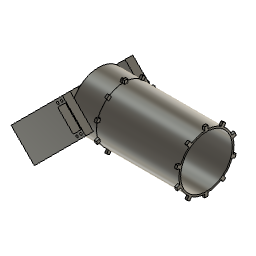
Cannon (Autodesk Fusion 360 archive; units mm, degrees)
design "Cannon" references "FeeTech FS5109M Metal Gear Servo Outer volume", "mg995"
Autodesk Fusion 360 part; units mm, degrees
sketch "Sketch1" plane through (0, 0, 0) normal (1, 0, 0) x (0, 1, 0)
  circle A0 centre (0, 0) radius 50
  circle A1 centre (0, 0) radius 47
  dimension "d1" = 94
  constraint coincident A0.centre A1.centre
  measures "d1" diameter of A1
extrude "Extrude1" add sketch "Sketch1" along normal blind 150 makes body 1
sketch "Sketch2" plane through (150, 0, 0) normal (1, 0, 0) x (0, 1, 0)
  circle A0 centre (0, 0) radius 47
  circle A1 centre (0, 0) radius 50
  line L0 (3, 49.9099) -> (-3, 49.9099)
  line L1 (-3, 49.9099) -> (-3, 55.9099)
  line L2 (-3, 55.9099) -> (3, 55.9099)
  line L3 (3, 55.9099) -> (3, 49.9099)
  line L4 (-35.2901, 43.4687) -> (-30.436, 46.9954)
  line L5 (-31.7634, 38.6146) -> (-35.2901, 43.4687)
  line L6 (-26.9093, 42.1413) -> (-31.7634, 38.6146)
  line L7 (-30.436, 46.9954) -> (-26.9093, 42.1413)
  line L8 (-54.1005, 14.4239) -> (-52.2464, 20.1303)
  line L9 (-48.3942, 12.5698) -> (-54.1005, 14.4239)
  line L10 (-46.5401, 18.2762) -> (-48.3942, 12.5698)
  line L11 (-52.2464, 20.1303) -> (-46.5401, 18.2762)
  line L12 (-52.2464, -20.1303) -> (-54.1005, -14.4239)
  line L13 (-46.5401, -18.2762) -> (-52.2464, -20.1303)
  line L14 (-48.3942, -12.5698) -> (-46.5401, -18.2762)
  line L15 (-54.1005, -14.4239) -> (-48.3942, -12.5698)
  line L16 (-30.436, -46.9954) -> (-35.2901, -43.4687)
  line L17 (-26.9093, -42.1413) -> (-30.436, -46.9954)
  line L18 (-31.7634, -38.6146) -> (-26.9093, -42.1413)
  line L19 (-35.2901, -43.4687) -> (-31.7634, -38.6146)
  line L20 (3, -55.9099) -> (-3, -55.9099)
  line L21 (3, -49.9099) -> (3, -55.9099)
  line L22 (-3, -49.9099) -> (3, -49.9099)
  line L23 (-3, -55.9099) -> (-3, -49.9099)
  line L24 (35.2901, -43.4687) -> (30.436, -46.9954)
  line L25 (31.7634, -38.6146) -> (35.2901, -43.4687)
  line L26 (26.9093, -42.1413) -> (31.7634, -38.6146)
  line L27 (30.436, -46.9954) -> (26.9093, -42.1413)
  line L28 (54.1005, -14.4239) -> (52.2464, -20.1303)
  line L29 (48.3942, -12.5698) -> (54.1005, -14.4239)
  line L30 (46.5401, -18.2762) -> (48.3942, -12.5698)
  line L31 (52.2464, -20.1303) -> (46.5401, -18.2762)
  line L32 (52.2464, 20.1303) -> (54.1005, 14.4239)
  line L33 (46.5401, 18.2762) -> (52.2464, 20.1303)
  line L34 (48.3942, 12.5698) -> (46.5401, 18.2762)
  line L35 (54.1005, 14.4239) -> (48.3942, 12.5698)
  line L36 (30.436, 46.9954) -> (35.2901, 43.4687)
  line L37 (26.9093, 42.1413) -> (30.436, 46.9954)
  line L38 (31.7634, 38.6146) -> (26.9093, 42.1413)
  line L39 (35.2901, 43.4687) -> (31.7634, 38.6146)
  dimension "d4" = 6
  dimension "d5" = 6
  dimension "d7" = 360
  constraint horizontal L0
  constraint vertical L1
  constraint horizontal L2
  constraint vertical L3
  constraint coincident A1 L0.start
  measures "d4" distance of L0.start L0.end
  measures "d5" distance of L0.start L2.end
extrude "Extrude2" add sketch "Sketch2" against normal blind 4 contours A1 L32 L33 L35 | A1 L28 L29 L31 | A1 L36 L37 L39 | A1 L24 L25 L27 | A1 L1 L2 L3 | A1 L20 L21 L23 | A1 L4 L5 L7 | A1 L16 L17 L19 | A1 L8 L9 L11 | A1 L12 L13 L15 bodies 1
sketch "Sketch3" plane through (0, 0, 0) normal (-1, 0, 0) x (0, -1, 0)
  circle A0 centre (0, 0) radius 47
  circle A1 centre (0, 0) radius 50
  line L0 (3, 49.9099) -> (-3, 49.9099)
  line L1 (-3, 49.9099) -> (-3, 55.9099)
  line L2 (-3, 55.9099) -> (3, 55.9099)
  line L3 (3, 55.9099) -> (3, 49.9099)
  line L4 (-35.2901, 43.4687) -> (-30.436, 46.9954)
  line L5 (-31.7634, 38.6146) -> (-35.2901, 43.4687)
  line L6 (-26.9093, 42.1413) -> (-31.7634, 38.6146)
  line L7 (-30.436, 46.9954) -> (-26.9093, 42.1413)
  line L8 (-54.1005, 14.4239) -> (-52.2464, 20.1303)
  line L9 (-48.3942, 12.5698) -> (-54.1005, 14.4239)
  line L10 (-46.5401, 18.2762) -> (-48.3942, 12.5698)
  line L11 (-52.2464, 20.1303) -> (-46.5401, 18.2762)
  line L12 (-52.2464, -20.1303) -> (-54.1005, -14.4239)
  line L13 (-46.5401, -18.2762) -> (-52.2464, -20.1303)
  line L14 (-48.3942, -12.5698) -> (-46.5401, -18.2762)
  line L15 (-54.1005, -14.4239) -> (-48.3942, -12.5698)
  line L16 (-30.436, -46.9954) -> (-35.2901, -43.4687)
  line L17 (-26.9093, -42.1413) -> (-30.436, -46.9954)
  line L18 (-31.7634, -38.6146) -> (-26.9093, -42.1413)
  line L19 (-35.2901, -43.4687) -> (-31.7634, -38.6146)
  line L20 (3, -55.9099) -> (-3, -55.9099)
  line L21 (3, -49.9099) -> (3, -55.9099)
  line L22 (-3, -49.9099) -> (3, -49.9099)
  line L23 (-3, -55.9099) -> (-3, -49.9099)
  line L24 (35.2901, -43.4687) -> (30.436, -46.9954)
  line L25 (31.7634, -38.6146) -> (35.2901, -43.4687)
  line L26 (26.9093, -42.1413) -> (31.7634, -38.6146)
  line L27 (30.436, -46.9954) -> (26.9093, -42.1413)
  line L28 (54.1005, -14.4239) -> (52.2464, -20.1303)
  line L29 (48.3942, -12.5698) -> (54.1005, -14.4239)
  line L30 (46.5401, -18.2762) -> (48.3942, -12.5698)
  line L31 (52.2464, -20.1303) -> (46.5401, -18.2762)
  line L32 (52.2464, 20.1303) -> (54.1005, 14.4239)
  line L33 (46.5401, 18.2762) -> (52.2464, 20.1303)
  line L34 (48.3942, 12.5698) -> (46.5401, 18.2762)
  line L35 (54.1005, 14.4239) -> (48.3942, 12.5698)
  line L36 (30.436, 46.9954) -> (35.2901, 43.4687)
  line L37 (26.9093, 42.1413) -> (30.436, 46.9954)
  line L38 (31.7634, 38.6146) -> (26.9093, 42.1413)
  line L39 (35.2901, 43.4687) -> (31.7634, 38.6146)
  dimension "d10" = 6
  dimension "d12" = 360
  constraint horizontal L0
  constraint vertical L1
  constraint horizontal L2
  constraint vertical L3
  constraint coincident A1 L0.start
  measures "d10" distance of L0.start L2.end
extrude "Extrude3" add sketch "Sketch3" against normal blind 4 contours A1 L32 L33 L35 | A1 L28 L29 L31 | A1 L36 L37 L39 | A1 L24 L25 L27 | A1 L1 L2 L3 | A1 L20 L21 L23 | A1 L4 L5 L7 | A1 L16 L17 L19 | A1 L8 L9 L11 | A1 L12 L13 L15 bodies 1
extrude "Extrude4" add sketch "Sketch1" along normal blind 3 contours A1 bodies 1
extrude "Extrude5" add sketch "Sketch1" against normal blind 60 separate body makes body 2
sketch "Sketch4" plane through (0, 0, 0) normal (-1, 0, 0) x (0, -1, 0)
  arc A0 (-46.5401, -18.2762) -> (-31.7634, -38.6146) centre (0, 0) ccw
  line L0 (-31.7634, -38.6146) -> (-35.2901, -43.4687)
  line L1 (-35.2901, -43.4687) -> (-30.436, -46.9954)
  line L2 (-30.436, -46.9954) -> (-26.9093, -42.1413)
  arc A1 (-26.9093, -42.1413) -> (-3, -49.9099) centre (0, 0) ccw
  line L3 (-3, -49.9099) -> (-3, -55.9099)
  line L4 (-3, -55.9099) -> (3, -55.9099)
  line L5 (3, -55.9099) -> (3, -49.9099)
  arc A2 (3, -49.9099) -> (26.9093, -42.1413) centre (0, 0) ccw
  line L6 (26.9093, -42.1413) -> (30.436, -46.9954)
  line L7 (30.436, -46.9954) -> (35.2901, -43.4687)
  line L8 (35.2901, -43.4687) -> (31.7634, -38.6146)
  arc A3 (31.7634, -38.6146) -> (46.5401, -18.2762) centre (0, 0) ccw
  line L9 (46.5401, -18.2762) -> (52.2464, -20.1303)
  line L10 (52.2464, -20.1303) -> (54.1005, -14.4239)
  line L11 (54.1005, -14.4239) -> (48.3942, -12.5698)
  arc A4 (48.3942, -12.5698) -> (48.3942, 12.5698) centre (0, 0) ccw
  line L12 (48.3942, 12.5698) -> (54.1005, 14.4239)
  line L13 (54.1005, 14.4239) -> (52.2464, 20.1303)
  line L14 (52.2464, 20.1303) -> (46.5401, 18.2762)
  arc A5 (46.5401, 18.2762) -> (31.7634, 38.6146) centre (0, 0) ccw
  line L15 (31.7634, 38.6146) -> (35.2901, 43.4687)
  line L16 (35.2901, 43.4687) -> (30.436, 46.9954)
  line L17 (30.436, 46.9954) -> (26.9093, 42.1413)
  arc A6 (26.9093, 42.1413) -> (3, 49.9099) centre (0, 0) ccw
  line L18 (3, 49.9099) -> (3, 55.9099)
  line L19 (3, 55.9099) -> (-3, 55.9099)
  line L20 (-3, 55.9099) -> (-3, 49.9099)
  arc A7 (-3, 49.9099) -> (-26.9093, 42.1413) centre (0, 0) ccw
  line L21 (-26.9093, 42.1413) -> (-30.436, 46.9954)
  line L22 (-30.436, 46.9954) -> (-35.2901, 43.4687)
  line L23 (-35.2901, 43.4687) -> (-31.7634, 38.6146)
  arc A8 (-31.7634, 38.6146) -> (-46.5401, 18.2762) centre (0, 0) ccw
  line L24 (-46.5401, 18.2762) -> (-52.2464, 20.1303)
  line L25 (-52.2464, 20.1303) -> (-54.1005, 14.4239)
  line L26 (-54.1005, 14.4239) -> (-48.3942, 12.5698)
  arc A9 (-48.3942, 12.5698) -> (-48.3942, -12.5698) centre (0, 0) ccw
  line L27 (-48.3942, -12.5698) -> (-54.1005, -14.4239)
  line L28 (-54.1005, -14.4239) -> (-52.2464, -20.1303)
  line L29 (-52.2464, -20.1303) -> (-46.5401, -18.2762)
  line L30 (-3, 49.9099) -> (0, 55.9099)
  line L31 (0, 55.9099) -> (3, 49.9099)
  line L32 (3, 49.9099) -> (-3, 49.9099)
  constraint coincident L20.end A7.start
  constraint midpoint L19 L30.end
  constraint coincident A6.end L18.start
move_body "Move1" bodies 1 to x (1, 0, 0) y (0, 1, 0) z (0, 0, 1) at (0, 0, -90)
extrude "Extrude6" add sketch "Sketch4" along normal blind 4 contours L30 L31 L32 bodies 2
move_body "Move2" bodies 1 to x (1, 0, 0) y (0, 1, 0) z (0, 0, 1) at (0, 0, 90)
sketch "Sketch5" plane through (0, 0, 0) normal (-1, 0, 0) x (0, -1, 0)
  arc A0 (-46.5401, -18.2762) -> (-31.7634, -38.6146) centre (0, 0) ccw
  line L0 (-31.7634, -38.6146) -> (-35.2901, -43.4687)
  line L1 (-35.2901, -43.4687) -> (-30.436, -46.9954)
  line L2 (-30.436, -46.9954) -> (-26.9093, -42.1413)
  arc A1 (-26.9093, -42.1413) -> (-3, -49.9099) centre (0, 0) ccw
  line L3 (-3, -49.9099) -> (-3, -55.9099)
  line L4 (-3, -55.9099) -> (3, -55.9099)
  line L5 (3, -55.9099) -> (3, -49.9099)
  arc A2 (3, -49.9099) -> (26.9093, -42.1413) centre (0, 0) ccw
  line L6 (26.9093, -42.1413) -> (30.436, -46.9954)
  line L7 (30.436, -46.9954) -> (35.2901, -43.4687)
  line L8 (35.2901, -43.4687) -> (31.7634, -38.6146)
  arc A3 (31.7634, -38.6146) -> (46.5401, -18.2762) centre (0, 0) ccw
  line L9 (46.5401, -18.2762) -> (52.2464, -20.1303)
  line L10 (52.2464, -20.1303) -> (54.1005, -14.4239)
  line L11 (54.1005, -14.4239) -> (48.3942, -12.5698)
  arc A4 (48.3942, -12.5698) -> (48.3942, 12.5698) centre (0, 0) ccw
  line L12 (48.3942, 12.5698) -> (54.1005, 14.4239)
  line L13 (54.1005, 14.4239) -> (52.2464, 20.1303)
  line L14 (52.2464, 20.1303) -> (46.5401, 18.2762)
  arc A5 (46.5401, 18.2762) -> (31.7634, 38.6146) centre (0, 0) ccw
  line L15 (31.7634, 38.6146) -> (35.2901, 43.4687)
  line L16 (35.2901, 43.4687) -> (30.436, 46.9954)
  line L17 (30.436, 46.9954) -> (26.9093, 42.1413)
  arc A6 (26.9093, 42.1413) -> (3, 49.9099) centre (0, 0) ccw
  line L18 (3, 49.9099) -> (3, 55.9099)
  line L19 (3, 55.9099) -> (-3, 55.9099)
  line L20 (-3, 55.9099) -> (-3, 49.9099)
  arc A7 (-3, 49.9099) -> (-26.9093, 42.1413) centre (0, 0) ccw
  line L21 (-26.9093, 42.1413) -> (-30.436, 46.9954)
  line L22 (-30.436, 46.9954) -> (-35.2901, 43.4687)
  line L23 (-35.2901, 43.4687) -> (-31.7634, 38.6146)
  arc A8 (-31.7634, 38.6146) -> (-46.5401, 18.2762) centre (0, 0) ccw
  line L24 (-46.5401, 18.2762) -> (-52.2464, 20.1303)
  line L25 (-52.2464, 20.1303) -> (-54.1005, 14.4239)
  line L26 (-54.1005, 14.4239) -> (-48.3942, 12.5698)
  arc A9 (-48.3942, 12.5698) -> (-48.3942, -12.5698) centre (0, 0) ccw
  line L27 (-48.3942, -12.5698) -> (-54.1005, -14.4239)
  line L28 (-54.1005, -14.4239) -> (-52.2464, -20.1303)
  line L29 (-52.2464, -20.1303) -> (-46.5401, -18.2762)
  circle A10 centre (0, 0) radius 1.5
  dimension "d27" = 3
  constraint coincident A0.centre A1.centre
  measures "d27" diameter of A10
extrude "Extrude7" cut sketch "Sketch5" against normal blind 1 contours A10 bodies 1
sketch "Sketch6" plane through (-41.4, 0, 0) normal (-1, 0, 0) x (0, -1, 0)
  line L0 (-6.05, 9.55) -> (-6.05, 7.55)
  arc A0 (-7.55, 6.05) -> (-6.05, 7.55) centre (-7.55, 7.55) ccw
  line L1 (-7.55, 6.05) -> (-9.55, 6.05)
  line L2 (-9.55, 6.05) -> (-9.55, -26.75)
  line L3 (-9.55, -26.75) -> (-7.55, -26.75)
  arc A1 (-6.05, -28.25) -> (-7.55, -26.75) centre (-7.55, -28.25) ccw
  line L4 (-6.05, -28.25) -> (-6.05, -30.25)
  line L5 (-6.05, -30.25) -> (6.05, -30.25)
  line L6 (6.05, -30.25) -> (6.05, -28.25)
  arc A2 (7.55, -26.75) -> (6.05, -28.25) centre (7.55, -28.25) ccw
  line L7 (7.55, -26.75) -> (9.55, -26.75)
  line L8 (9.55, -26.75) -> (9.55, 6.05)
  line L9 (9.55, 6.05) -> (7.55, 6.05)
  arc A3 (6.05, 7.55) -> (7.55, 6.05) centre (7.55, 7.55) ccw
  line L10 (6.05, 7.55) -> (6.05, 9.55)
  line L11 (6.05, 9.55) -> (-6.05, 9.55)
  line L12 (-90, 80) -> (102.9005, 80)
  line L13 (102.9005, 80) -> (102.9005, -93.0989)
  line L14 (102.9005, -93.0989) -> (-90, -93.0989)
  line L15 (-90, -93.0989) -> (-90, 80)
  constraint horizontal L12
  constraint vertical L13
  constraint horizontal L14
  constraint vertical L15
extrude "Extrude8" cut sketch "Sketch6" against normal blind 280 keep common part bodies 1 2
move_body "Move3" bodies 1 to x (1, 0, 0) y (0, 1, 0) z (0, 0, 1) at (0, 0, 115)
move_body "Move4" bodies 1 to x (1, 0, 0) y (0, 1, 0) z (0, 0, 1) at (0, 0, -115)
extrude "Extrude9" add sketch "Sketch1" along normal blind 3 contours A1 bodies 1
extrude "Extrude10" cut sketch "Sketch5" against normal blind 1 contours A10 bodies 1
extrude "Extrude11" add 1 faces at (-41.4, 48.8138, -2.484) along direction (-1, 0, 0) blind 5 on bodies 2 bodies 2
sketch "Sketch7" plane through (-46.4, 0, 0) normal (-1, 0, 0) x (0, -1, 0)
  circle A0 centre (0, 0) radius 47
  circle A1 centre (0, 0) radius 50
  circle A2 centre (0, 0) radius 47
  constraint coincident A0.centre A1.centre
extrude "Extrude12" add sketch "Sketch7" against normal blind 4 contours A0 A2 bodies 2
sketch "Sketch8" plane through (-46.4, 0, 0) normal (-1, 0, 0) x (0, -1, 0)
  circle A0 centre (0, 0) radius 50
  line L0 (-40, 20) -> (-25, 20)
  line L1 (-25, 20) -> (-25, -20)
  line L2 (-25, -20) -> (-40, -20)
  line L3 (-40, -20) -> (-40, 20)
  dimension "d50" = 15
  dimension "d51" = 40
  constraint horizontal L0
  constraint vertical L1
  constraint horizontal L2
  constraint vertical L3
  measures "d50" distance of L0.start L0.end
  measures "d51" distance of L0.start L2.end
extrude "Extrude13" cut sketch "Sketch8" against normal blind 10 contours L0 L1 L2 L3 bodies 2
sketch "Sketch9" plane through (-14.6, 0, 0) normal (-1, 0, 0) x (0, -1, 0)
  arc A0 (9.35, 9.8189) -> (8.55, 10.05) centre (8.55, 8.55) ccw
  line L0 (9.35, 9.8189) -> (9.35, 15.45)
  arc A1 (9.35, 15.45) -> (7.85, 16.95) centre (7.85, 15.45) ccw
  line L1 (7.85, 16.95) -> (6.25, 16.95)
  line L2 (6.25, 16.95) -> (6.25, 16.2708)
  arc A2 (3.75, 16.2708) -> (6.25, 16.2708) centre (5, 14.4) ccw
  line L3 (3.75, 16.2708) -> (3.75, 16.95)
  line L4 (3.75, 16.95) -> (-3.75, 16.95)
  line L5 (-3.75, 16.95) -> (-3.75, 16.2708)
  arc A3 (-6.25, 16.2708) -> (-3.75, 16.2708) centre (-5, 14.4) ccw
  line L6 (-6.25, 16.2708) -> (-6.25, 16.95)
  line L7 (-6.25, 16.95) -> (-7.85, 16.95)
  arc A4 (-7.85, 16.95) -> (-9.35, 15.45) centre (-7.85, 15.45) ccw
  line L8 (-9.35, 15.45) -> (-9.35, 9.8189)
  arc A5 (-8.55, 10.05) -> (-9.35, 9.8189) centre (-8.55, 8.55) ccw
  line L9 (-8.55, 10.05) -> (8.55, 10.05)
  line L10 (-9.35, 10.9766) -> (9.35, 10.9766)
  line L11 (9.35, 10.9766) -> (9.35, 69.9703)
  line L12 (9.35, 69.9703) -> (-9.35, 69.9703)
  line L13 (-9.35, 69.9703) -> (-9.35, 10.9766)
  line L14 (-9.35, -31.9165) -> (9.35, -31.9165)
  line L15 (9.35, -31.9165) -> (9.35, -86.2684)
  line L16 (9.35, -86.2684) -> (-9.35, -86.2684)
  line L17 (-9.35, -86.2684) -> (-9.35, -31.9165)
  circle A6 centre (-5, 14.4) radius 2.25
  circle A7 centre (5, 14.4) radius 2.25
  circle A8 centre (5, -35) radius 2.2361
  circle A9 centre (-5, -35) radius 2.2361
  constraint horizontal L10
  constraint vertical L11
  constraint horizontal L12
  constraint vertical L13
  constraint coincident L8 L10.start
  constraint horizontal L14
  constraint vertical L15
  constraint horizontal L16
  constraint vertical L17
  constraint concentric A3 A6
  constraint concentric A2 A7
extrude "Extrude14" add sketch "Sketch9" along normal blind 5 contours L0 A1 L1 L2 A2 L3 L4 L5 A3 L6 L7 A4 L8 L10 L11 L13 A6 A7 | A1 L1 L2 L3 L4 L5 L6 L7 A4 L11 L12 L13 A6 A7 | L14 L15 L16 L17 bodies 2
extrude "Extrude15" cut 2 faces at (-14.6, 1.0444, 63.2808) (-14.6, 1.0444, -74.1462) along direction (-1, 0, 0) blind 10 on bodies 2 bodies 2
ref_plane "WorkPlane1" through (0, -50, 0) normal (0, 1, 0) x (0, 0, 1)
sketch "Sketch10" plane through (0, -50, 0) normal (0, 1, 0) x (1, 0, 0)
  line L0 (0, 0) -> (-42.4264, -42.4264)
  line L1 (0, 0) -> (60, 0) construction
  line L2 (-42.4264, -42.4264) -> (-148.4924, 63.6396)
  line L3 (-148.4924, 63.6396) -> (-106.066, 106.066)
  line L4 (-106.066, 106.066) -> (0, 0)
  circle A0 centre (-28.2843, 0) radius 1
  point P0 (-28.2843, 0)
  dimension "d59" = 135
  dimension "d60" = 60
  dimension "d61" = 150
  dimension "d62" = 60
  dimension "d81" = 2
  constraint horizontal L1
  constraint coincident L0.start L1.start
  constraint perpendicular L0 L2
  constraint perpendicular L2 L3
  constraint coincident P0 A0.centre
  measures "d59" angle of L0 L1
  measures "d60" distance of L0.start L0.end
  measures "d61" distance of L0.end L2.end
  measures "d62" distance of L2.end L3.end
  measures "d81" diameter of A0
extrude "Extrude16" add sketch "Sketch10" against normal blind 14 separate body contours L0 L2 L3 L4 | A0 makes body 3
sketch "Sketch11" plane through (0, -58, 0) normal (0, 1, 0) x (-1, 0, 0)
  arc A0 (25.0025, 9.4462) -> (21.2132, 7.0711) centre (28.2843, 0) ccw
  line L0 (25.0025, 9.4462) -> (39.2444, 23.6881)
  line L1 (39.2444, 23.6881) -> (51.9723, 10.9602)
  line L2 (51.9723, 10.9602) -> (37.7304, -3.2818)
  arc A1 (35.3553, -7.0711) -> (37.7304, -3.2818) centre (28.2843, 0) ccw
  line L3 (35.3553, -7.0711) -> (56.5685, 14.1421)
  line L4 (56.5685, 14.1421) -> (42.4264, 28.2843)
  line L5 (42.4264, 28.2843) -> (21.2132, 7.0711)
sketch "Sketch12" plane through (0, -58, 0) normal (0, 1, 0) x (-1, 0, 0)
  line L0 (42.4264, 28.2841) -> (14.1421, -0.0002)
  line L1 (42.4264, 28.2841) -> (82.4264, 28.2841) construction
  line L2 (14.1421, -0.0002) -> (28.2842, -14.1423)
  line L3 (28.2842, -14.1423) -> (56.5685, 14.142)
  line L4 (56.5685, 14.142) -> (42.4264, 28.2841)
  dimension "d70" = 135
  dimension "d71" = 40
  constraint horizontal L1
  constraint perpendicular L0 L2
  constraint perpendicular L2 L3
  constraint perpendicular L0 L4
  measures "d70" angle of L0 L1
  measures "d71" distance of L0.start L0.end
extrude "Extrude17" cut sketch "Sketch12" along normal blind 10 and the other way blind 9 bodies 3
sketch "Sketch13" plane through (0, -66.5, 0) normal (0, -1, 0) x (1, 0, 0)
  arc A0 (-51.4134, 28.786) -> (-49.9992, 30.2002) centre (-49.3207, 28.1075) ccw
  line L0 (-51.4134, 28.786) -> (-51.6188, 28.9914)
  line L1 (-51.6188, 28.9914) -> (-57.2756, 23.3345)
  line L2 (-57.2756, 23.3345) -> (-57.0703, 23.1292)
  arc A1 (-58.4845, 21.715) -> (-57.0703, 23.1292) centre (-56.3918, 21.0364) ccw
  line L3 (-58.4845, 21.715) -> (-58.6899, 21.9203)
  line L4 (-58.6899, 21.9203) -> (-61.5183, 19.0919)
  line L5 (-61.5183, 19.0919) -> (-56.5685, 14.1421)
  line L6 (-56.5685, 14.1421) -> (-42.4264, 28.2843)
  line L7 (-42.4264, 28.2843) -> (-47.3762, 33.234)
  line L8 (-47.3762, 33.234) -> (-50.2046, 30.4056)
  line L9 (-50.2046, 30.4056) -> (-49.9992, 30.2002)
  circle A2 centre (-49.3207, 28.1075) radius 2.2
  circle A3 centre (-56.3918, 21.0364) radius 2.2
  line L10 (-17.6815, -3.5317) -> (-14.3227, -6.8905)
  circle A4 centre (-14.3227, -6.8905) radius 2.2
  circle A5 centre (-21.3938, -13.9615) radius 2.2
  dimension "d76" = 4.75
  dimension "d77" = 4.4
  dimension "d78" = 4.4
  constraint concentric A0 A2
  constraint concentric A1 A3
  constraint coincident L10.end A4.centre
  measures "d76" distance of L10.start L10.end
  measures "d77" diameter of A4
  measures "d78" diameter of A5
extrude "Extrude18" cut sketch "Sketch13" against normal blind 30 contours A0 A2 | A1 A3 | A4 | A5 bodies 3
extrude "Extrude19" cut sketch "Sketch10" along normal blind 1 contours A0 bodies 2
sketch "Sketch14" plane through (0, -50, 0) normal (0, 1, 0) x (-1, 0, 0)
  circle A0 centre (56.3918, 21.0364) radius 2.2
  circle A1 centre (14.3227, -6.8905) radius 2.2
  circle A2 centre (49.3207, 28.1075) radius 2.2
  circle A3 centre (21.3938, -13.9615) radius 2.2
  line L0 (106.066, -106.066) -> (148.4924, -63.6396)
  line L1 (148.4924, -63.6396) -> (42.4264, 42.4264)
  line L2 (42.4264, 42.4264) -> (0, 0)
  line L3 (0, 0) -> (106.066, -106.066)
  line L4 (134.3503, -49.4975) -> (91.9239, -91.9239)
  line L5 (56.5685, 14.142) -> (28.2842, -14.1423)
  line L6 (28.2842, -14.1423) -> (14.1421, -0.0002)
  line L7 (14.1421, -0.0002) -> (42.4264, 28.2841)
  line L8 (42.4264, 28.2841) -> (56.5685, 14.142)
  dimension "d84" = 20
  constraint coincident L3 L4.end
  constraint perpendicular L3 L4
  measures "d84" distance of L0.end L4.start
extrude "Extrude20" add sketch "Sketch14" along normal blind 114 contours L0 L1 L3 L4 bodies 3
sketch "Sketch15" plane through (-91.9239, 0, -91.9239) normal (0.707107, 0, 0.707107) x (0, 1, 0)
  line L0 (-50, 60) -> (-50, 0)
  line L1 (-50, 0) -> (64, 0)
  line L2 (64, 0) -> (64, 60)
  line L3 (64, 60) -> (-50, 60)
  line L4 (50, 0) -> (50, 60)
  dimension "d87" = 14
  constraint coincident L3 L4.end
  constraint perpendicular L3 L4
  measures "d87" distance of L1.end L4.start
extrude "Extrude21" add sketch "Sketch15" along normal blind 122 contours L1 L2 L3 L4 bodies 3
move_face "OffsetFaces1" offset -8 1 faces at (-14.1421, -54.6667, 14.1421) on bodies 3
ref_plane "WorkPlane2" through (0, 50, 0) normal (0, 1, 0) x (0, 0, 1)
sketch "Sketch16" plane through (0, 50, 0) normal (0, 1, 0) x (1, 0, 0)
  circle A0 centre (-28.2, 0) radius 5
  dimension "d92" = 28.2
  dimension "d93" = 10
  measures "d92" distance of origin A0.centre
  measures "d93" diameter of A0
extrude "Extrude22" cut sketch "Sketch16" along normal blind 20 and the other way blind 10 bodies 2 3
sketch "Sketch17" plane through (-91.9239, 0, -91.9239) normal (0.707107, 0, 0.707107) x (0, 1, 0)
  line L0 (50, 0) -> (50, 60)
  line L1 (50, 60) -> (-50, 60)
  line L2 (-50, 60) -> (-50, 0)
  line L3 (-50, 0) -> (50, 0)
move_face "OffsetFaces2" offset -10 1 faces at (-120.2082, -21.3333, -91.9239) on bodies 3
sketch "Sketch18" plane through (-91.9239, 0, -91.9239) normal (0.707107, 0, 0.707107) x (0, 1, 0)
  circle A0 centre (-30, 50) radius 1.9
  circle A1 centre (0, 50) radius 1.9
  circle A2 centre (30, 50) radius 1.9
  circle A3 centre (-30, 10) radius 1.9
  circle A4 centre (0, 10) radius 1.9
  circle A5 centre (30, 10) radius 1.9
  dimension "d99" = 3.8
  dimension "d100" = 3.8
  dimension "d101" = 3.8
  dimension "d102" = 3.8
  dimension "d103" = 3.8
  dimension "d104" = 3.8
  measures "d99" diameter of A0
  measures "d100" diameter of A1
  measures "d101" diameter of A2
  measures "d102" diameter of A3
  measures "d103" diameter of A4
  measures "d104" diameter of A5
extrude "Extrude23" cut sketch "Sketch18" against normal blind 40 bodies 3
copy_body "Body->Comp1" bodies 1 removing the originals makes body 4 in component "Barrel"
copy_body "Body->Comp2" bodies 2 removing the originals makes body 5 in component "Base"
copy_body "Body->Comp3" bodies 3 removing the originals makes body 6 in component "Support"
move_face "OffsetFaces1'" offset -2 2 faces at (-14.6, -1.0317, 26.6651) (-14.6, 1.0451, -40.1306) on bodies 5 in component "Base"
sketch "Sketch19" plane through (0, 0, 0) normal (-1, 0, 0) x (0, -1, 0)
  circle A0 centre (0, 0) radius 1.5
  arc A1 (-46.5401, -18.2762) -> (-31.7634, -38.6146) centre (0, 0) ccw
  line L0 (-31.7634, -38.6146) -> (-35.2901, -43.4687)
  line L1 (-35.2901, -43.4687) -> (-30.436, -46.9954)
  line L2 (-30.436, -46.9954) -> (-26.9093, -42.1413)
  arc A2 (-26.9093, -42.1413) -> (-3, -49.9099) centre (0, 0) ccw
  line L3 (-3, -49.9099) -> (-3, -55.9099)
  line L4 (-3, -55.9099) -> (3, -55.9099)
  line L5 (3, -55.9099) -> (3, -49.9099)
  arc A3 (3, -49.9099) -> (26.9093, -42.1413) centre (0, 0) ccw
  line L6 (26.9093, -42.1413) -> (30.436, -46.9954)
  line L7 (30.436, -46.9954) -> (35.2901, -43.4687)
  line L8 (35.2901, -43.4687) -> (31.7634, -38.6146)
  arc A4 (31.7634, -38.6146) -> (46.5401, -18.2762) centre (0, 0) ccw
  line L9 (46.5401, -18.2762) -> (52.2464, -20.1303)
  line L10 (52.2464, -20.1303) -> (54.1005, -14.4239)
  line L11 (54.1005, -14.4239) -> (48.3942, -12.5698)
  arc A5 (48.3942, -12.5698) -> (48.3942, 12.5698) centre (0, 0) ccw
  line L12 (48.3942, 12.5698) -> (54.1005, 14.4239)
  line L13 (54.1005, 14.4239) -> (52.2464, 20.1303)
  line L14 (52.2464, 20.1303) -> (46.5401, 18.2762)
  arc A6 (46.5401, 18.2762) -> (31.7634, 38.6146) centre (0, 0) ccw
  line L15 (31.7634, 38.6146) -> (35.2901, 43.4687)
  line L16 (35.2901, 43.4687) -> (30.436, 46.9954)
  line L17 (30.436, 46.9954) -> (26.9093, 42.1413)
  arc A7 (26.9093, 42.1413) -> (3, 49.9099) centre (0, 0) ccw
  line L18 (3, 49.9099) -> (3, 55.9099)
  line L19 (3, 55.9099) -> (-3, 55.9099)
  line L20 (-3, 55.9099) -> (-3, 49.9099)
  arc A8 (-3, 49.9099) -> (-26.9093, 42.1413) centre (0, 0) ccw
  line L21 (-26.9093, 42.1413) -> (-30.436, 46.9954)
  line L22 (-30.436, 46.9954) -> (-35.2901, 43.4687)
  line L23 (-35.2901, 43.4687) -> (-31.7634, 38.6146)
  arc A9 (-31.7634, 38.6146) -> (-46.5401, 18.2762) centre (0, 0) ccw
  line L24 (-46.5401, 18.2762) -> (-52.2464, 20.1303)
  line L25 (-52.2464, 20.1303) -> (-54.1005, 14.4239)
  line L26 (-54.1005, 14.4239) -> (-48.3942, 12.5698)
  arc A10 (-48.3942, 12.5698) -> (-48.3942, -12.5698) centre (0, 0) ccw
  line L27 (-48.3942, -12.5698) -> (-54.1005, -14.4239)
  line L28 (-54.1005, -14.4239) -> (-52.2464, -20.1303)
  line L29 (-52.2464, -20.1303) -> (-46.5401, -18.2762)
  circle A11 centre (0, 7) radius 1.5
  circle A12 centre (-7, 0) radius 1.5
  circle A13 centre (0, -7) radius 1.5
  circle A14 centre (7, 0) radius 1.5
  dimension "d108" = 3
  dimension "d110" = 360
  measures "d108" diameter of A11
extrude "Extrude1'" cut sketch "Sketch19" against normal blind 22 contours A11 | A12 | A13 | A14 bodies 4 in component "Barrel"
sketch "Sketch20" plane through (0, 0, 0) normal (-1, 0, 0) x (0, -1, 0)
  circle A0 centre (-7, 0) radius 1.5
  circle A1 centre (0, -7) radius 1.5
  circle A2 centre (0, 7) radius 1.5
  circle A3 centre (7, 0) radius 1.5
  circle A4 centre (0, 0) radius 1.5
  arc A5 (-46.5401, -18.2762) -> (-31.7634, -38.6146) centre (0, 0) ccw
  line L0 (-31.7634, -38.6146) -> (-35.2901, -43.4687)
  line L1 (-35.2901, -43.4687) -> (-30.436, -46.9954)
  line L2 (-30.436, -46.9954) -> (-26.9093, -42.1413)
  arc A6 (-26.9093, -42.1413) -> (-3, -49.9099) centre (0, 0) ccw
  line L3 (-3, -49.9099) -> (-3, -55.9099)
  line L4 (-3, -55.9099) -> (3, -55.9099)
  line L5 (3, -55.9099) -> (3, -49.9099)
  arc A7 (3, -49.9099) -> (26.9093, -42.1413) centre (0, 0) ccw
  line L6 (26.9093, -42.1413) -> (30.436, -46.9954)
  line L7 (30.436, -46.9954) -> (35.2901, -43.4687)
  line L8 (35.2901, -43.4687) -> (31.7634, -38.6146)
  arc A8 (31.7634, -38.6146) -> (46.5401, -18.2762) centre (0, 0) ccw
  line L9 (46.5401, -18.2762) -> (52.2464, -20.1303)
  line L10 (52.2464, -20.1303) -> (54.1005, -14.4239)
  line L11 (54.1005, -14.4239) -> (48.3942, -12.5698)
  arc A9 (48.3942, -12.5698) -> (48.3942, 12.5698) centre (0, 0) ccw
  line L12 (48.3942, 12.5698) -> (54.1005, 14.4239)
  line L13 (54.1005, 14.4239) -> (52.2464, 20.1303)
  line L14 (52.2464, 20.1303) -> (46.5401, 18.2762)
  arc A10 (46.5401, 18.2762) -> (31.7634, 38.6146) centre (0, 0) ccw
  line L15 (31.7634, 38.6146) -> (35.2901, 43.4687)
  line L16 (35.2901, 43.4687) -> (30.436, 46.9954)
  line L17 (30.436, 46.9954) -> (26.9093, 42.1413)
  arc A11 (26.9093, 42.1413) -> (3, 49.9099) centre (0, 0) ccw
  line L18 (3, 49.9099) -> (3, 55.9099)
  line L19 (3, 55.9099) -> (-3, 55.9099)
  line L20 (-3, 55.9099) -> (-3, 49.9099)
  arc A12 (-3, 49.9099) -> (-26.9093, 42.1413) centre (0, 0) ccw
  line L21 (-26.9093, 42.1413) -> (-30.436, 46.9954)
  line L22 (-30.436, 46.9954) -> (-35.2901, 43.4687)
  line L23 (-35.2901, 43.4687) -> (-31.7634, 38.6146)
  arc A13 (-31.7634, 38.6146) -> (-46.5401, 18.2762) centre (0, 0) ccw
  line L24 (-46.5401, 18.2762) -> (-52.2464, 20.1303)
  line L25 (-52.2464, 20.1303) -> (-54.1005, 14.4239)
  line L26 (-54.1005, 14.4239) -> (-48.3942, 12.5698)
  arc A14 (-48.3942, 12.5698) -> (-48.3942, -12.5698) centre (0, 0) ccw
  line L27 (-48.3942, -12.5698) -> (-54.1005, -14.4239)
  line L28 (-54.1005, -14.4239) -> (-52.2464, -20.1303)
  line L29 (-52.2464, -20.1303) -> (-46.5401, -18.2762)
extrude "Extrude2'" cut sketch "Sketch20" against normal blind 40 contours A4 bodies 4 in component "Barrel"
extrude "Extrude1''" cut sketch "Sketch16" against normal blind 120 bodies 5 in component "Base"
sketch "Sketch21" plane through (-42.4, 0, 0) normal (1, 0, 0) x (0, 1, 0)
  line L0 (25, -20) -> (25, 20)
  line L1 (25, 20) -> (40, 20)
  line L2 (40, 20) -> (40, -20)
  line L3 (40, -20) -> (25, -20)
  circle A0 centre (0, 0) radius 47
  line L4 (-47, 0) -> (-47, 4)
  line L5 (-47, 4) -> (47, 4)
  line L6 (47, 4) -> (47, -4)
  line L7 (47, -4) -> (-47, -4)
  line L8 (-47, -4) -> (-47, 4)
  point P0 (46.8295, 4)
  constraint coincident A0 L4.start
  constraint vertical L4
  constraint coincident A0 P0
  constraint horizontal L5
  constraint vertical L6
  constraint horizontal L7
  constraint vertical L8
extrude "Extrude1'''" add sketch "Sketch16" against normal blind 120 separate body makes body 7 in component "Shaft"
move_body "Move1'" bodies 7 to x (1, 0, 0) y (0, 1, 0) z (0, 0, 1) at (0, 15, 0) in component "Shaft"
extrude "Extrude2''" cut sketch "Sketch21" along normal blind 15 contours L0 A0 L5 L7 | L0 L2 L5 L7 | L2 A0 L5 L7 bodies 7 in component "Shaft"
move_body "Move2'" bodies 7 to x (1, 0, 0) y (0, 1, 0) z (0, 0, 1) at (0, 15, 0) in component "Shaft"
move_body "Move3'" bodies 7 to x (1, 0, 0) y (0, 1, 0) z (0, 0, 1) at (0, -10, 0) in component "Shaft"
extrude "Extrude3'" cut sketch "Sketch21" along normal blind 15 contours L0 A0 L5 L7 | L0 L2 L5 L7 | L2 A0 L5 L7 bodies 7 in component "Shaft"
extrude "Extrude2'''" add sketch "Sketch21" along normal blind 14 contours L0 A0 L5 L7 | L0 L2 L5 L7 | L2 A0 L5 L7 bodies 5 in component "Base"
move_body "Move4'" bodies 7 to x (1, 0, 0) y (0, 1, 0) z (0, 0, 1) at (0, -40, 0) in component "Shaft"
extrude "Extrude4'" cut sketch "Sketch21" along normal blind 15 contours L0 A0 L5 L7 | L0 L2 L5 L7 | L2 A0 L5 L7 bodies 7 in component "Shaft"
move_body "Move5" bodies 7 to x (1, 0, 0) y (0, 1, 0) z (0, 0, 1) at (0, 40, 0) in component "Shaft"
sketch "Sketch22" plane through (0, -50, 0) normal (0, -1, 0) x (1, 0, 0)
  circle A0 centre (-28.2, 0) radius 5
  circle A1 centre (-28.2, 0) radius 1.5
  dimension "d127" = 3
  constraint concentric A0 A1
  measures "d127" diameter of A1
extrude "Extrude5'" cut sketch "Sketch22" against normal blind 30 contours A1 bodies 7 in component "Shaft"
sketch "Sketch23" plane through (-27.4, 0, 0) normal (-1, 0, 0) x (0, -1, 0)
  line L0 (46.9829, -1.2689) -> (20, -1.2689)
  line L1 (20, -1.2689) -> (20, 1.2689)
  line L2 (20, 1.2689) -> (46.9829, 1.2689)
  arc A0 (46.9829, 1.2689) -> (46.8295, 4) centre (0, 0) ccw
  line L3 (46.8295, 4) -> (-70, 4)
  line L4 (-70, 4) -> (-70, -4)
  line L5 (-70, -4) -> (46.8295, -4)
  arc A1 (46.8295, -4) -> (46.9829, -1.2689) centre (0, 0) ccw
  line L6 (46.9829, 1.2689) -> (46.9829, 1.7689)
  line L7 (46.9829, -1.2689) -> (46.9829, -1.7689)
  line L8 (46.9829, 1.7689) -> (19.9929, 1.7689)
  line L9 (19.9929, 1.7689) -> (19.9929, -1.7689)
  line L10 (19.9929, -1.7689) -> (46.9829, -1.7689)
  line L11 (46.9829, -1.7689) -> (46.9829, 1.7689)
  dimension "d130" = 0.5
  dimension "d131" = 0.5
  constraint coincident L2.end A0.start
  constraint perpendicular L2 L6
  constraint coincident L0.start A1.end
  constraint perpendicular L5 L7
  constraint horizontal L8
  constraint vertical L9
  constraint horizontal L10
  constraint vertical L11
  measures "d130" distance of L2.end L6.end
  measures "d131" distance of L0.start L7.end
extrude "Extrude6'" cut sketch "Sketch23" against normal blind 1 contours L0 L1 L2 A0 A1 L8 L9 L10 | L0 L1 L2 L11 bodies 7 in component "Shaft"
component "Barrel" placed x (1, 0, 0) y (0, 1, 0) z (0, 0, 1) at (0, 0, 0)
component "Support" placed x (1, 0, 0) y (0, 1, 0) z (0, 0, 1) at (0, 0, 0)
component "Base" placed x (1, 0, 0) y (0, 1, 0) z (0, 0, 1) at (0, 0, 0)
component "Shaft" placed x (1, 0, 0) y (0, 1, 0) z (0, 0, 1) at (0, 0, 0)
